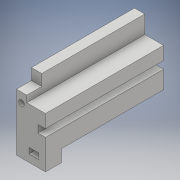
# Autodesk Inventor part: side
Saved by Autodesk Inventor 2018 (Build 220112000, 112)
## iProperties
Created: 2018-05-15
Part Number: side
Material: Generic
Document SubType Name: Modeling
Designer: bitbots
Density: 1 g/cm^3
Appearance: Default
Author: bitbots
Autodesk Inventor part; units mm, degrees
ref_plane "YZ Plane" through (0, 0, 0) normal (1, 0, 0) x (0, 1, 0)
ref_plane "XZ Plane" through (0, 0, 0) normal (0, 1, 0) x (-1, 0, 0)
ref_plane "XY Plane" through (0, 0, 0) normal (0, 0, 1) x (1, 0, 0)
ref_plane "Work Plane1" through (0, 0, 0) normal (0, 0, 1) x (1, 0, 0)
sketch "Sketch1" plane through (0, 0, 0) normal (0, 0, 1) x (1, 0, 0)
  circle A0 centre (-17.3, 4) radius 1.35 projected
  circle A1 centre (-17.3, -18) radius 1.35 projected
  circle A2 centre (-17.3, -40) radius 1.35 projected
  line L0 (-17.3, 4) -> (-14.8, 4)
  line L1 (-14.8, 4) -> (-14.8, 9)
  line L2 (-14.8, 9) -> (-20.3, 9)
  line L3 (-17.3, -40) -> (-17.3, -54)
  line L4 (-14.8, 4) -> (-14.8, -54)
  line L5 (-14.8, -54) -> (-17.3, -54)
  line L6 (-17.3, -54) -> (-20.3, -54)
  line L7 (-20.3, -54) -> (-20.3, 9)
  point P0 (0, 0)
  dimension "d0" = 2.5
  dimension "d1" = 5
  dimension "d2" = 5.5
  dimension "d3" = 14
  constraints: 16 end point, 3 perpendicular, 2 horizontal, 1 parallel, 1 point on line, 1 vertical
  measures "d0" distance of L0.start L0.end
  measures "d1" distance of L0.end L1.end
  measures "d2" distance of L1.end L2.end
  measures "d3" distance of L3.start L3.end
extrude "Extrusion1" add sketch "Sketch1" along normal blind 36.5
sketch "Sketch2" plane through (-20.3, -54, 0) normal (0, -1, 0) x (1, 0, 0)
  line L0 (0, 0) -> (5.5, 0) projected
  line L1 (5.5, 0) -> (5.5, 36.5) projected
  line L2 (0, 36.5) -> (5.5, 36.5) projected
  line L3 (0, 0) -> (0, 36.5) projected
  line L4 (2.75, 36.5) -> (2.75, 25.5)
  circle A0 centre (2.75, 25.5) radius 1.5
  point P0 (20.3, 0)
  dimension "d6" = 11
  dimension "d7" = 3
  constraints: 2 end point, 1 centre point, 1 coincident, 1 midpoint, 1 vertical
  measures "d6" distance of L4.start L4.end
  measures "d7" diameter of A0
extrude "Extrusion2" cut sketch "Sketch2" against normal blind 10 contours A0
sketch "Sketch3" plane through (-20.3, -54, 0) normal (-1, 0, 0) x (0, 0, 1)
  line L0 (0, 63) -> (0, 0) projected
  line L1 (0, 0) -> (36.5, 0) projected
  line L2 (36.5, 63) -> (36.5, 0) projected
  line L3 (0, 63) -> (36.5, 63) projected
  line L4 (0, 0) -> (36.5, 0) projected
  line L5 (36.5, 0) -> (28.5, 0)
  line L6 (28.5, 0) -> (28.5, 8)
  line L7 (28.5, 8) -> (36.5, 8)
  line L8 (36.5, 8) -> (36.5, 0)
  point P0 (0, 54)
  dimension "d10" = 8
  dimension "d11" = 8
  constraints: 8 end point, 2 parallel, 1 horizontal, 1 perpendicular
  measures "d10" distance of L6.end L7.end
  measures "d11" distance of L5.end L6.end
extrude "Extrusion3" cut sketch "Sketch3" against normal blind 10 contours L6 L7 L2 L1
sketch "Sketch4" plane through (-20.3, 9, 0) normal (0, 1, 0) x (1, 0, 0)
  line L0 (5.5, 0) -> (0, 0) projected
  line L1 (0, 0) -> (0, -36.5) projected
  line L2 (5.5, -36.5) -> (0, -36.5) projected
  line L3 (5.5, 0) -> (5.5, -36.5) projected
  line L4 (6.8, -6) -> (8.8, -6) projected
  line L5 (6.8, -6) -> (5.5, -6)
  line L6 (5.5, -6) -> (5.5, -6.5)
  line L7 (5.5, 0) -> (5.5, -28.5) projected
  line L8 (5.5, -6.5) -> (15.5, -6.5)
  line L9 (15.5, -6.5) -> (15.5, -11.5)
  line L10 (15.5, -11.5) -> (5.5, -11.5)
  line L11 (5.5, -11.5) -> (5.5, -6.5)
  point P0 (20.3, 0)
  dimension "d14" = 0.5
  dimension "d15" = 10
  dimension "d16" = 5
  constraints: 12 end point, 2 parallel, 2 perpendicular, 2 point on line, 1 horizontal
  measures "d14" distance of L5.end L6.end
  measures "d15" distance of L9.end L10.end
  measures "d16" distance of L8.end L9.end
extrude "Extrusion4" add sketch "Sketch4" against normal up to surface (63 mm away) contours L8 L9 L10 L3
sketch "Sketch5" plane through (-4.8, 9, 6.5) normal (0, 0, -1) x (-1, 0, 0)
  circle A0 centre (12.5, -49) radius 1.35 projected
  circle A1 centre (12.5, -27) radius 1.35 projected
  circle A2 centre (12.5, -5) radius 1.35 projected
  line L0 (10, -63) -> (10, 0) projected
  line L1 (15.5, -63) -> (10, -63) projected
  line L2 (15.5, 0) -> (15.5, -63) projected
  line L3 (10, 0) -> (15.5, 0) projected
  line L4 (0, -63) -> (10, -63) projected
  line L5 (10, 0) -> (10, -63) projected
  line L6 (0, 0) -> (10, 0) projected
  line L7 (0, 0) -> (0, -63) projected
  line L8 (-19.8, 5.5) -> (-16.3, 5.5) projected
  line L9 (-19.8, 5.5) -> (-24.9, -0.5) projected
  line L10 (-24.9, -0.5) -> (-24.9, -53.6) projected
  line L11 (-24.9, -53.6) -> (-19.8, -59.6) projected
  line L12 (-19.8, -59.6) -> (10.2, -59.6) projected
  line L13 (10.2, -59.6) -> (15.3, -53.6) projected
  line L14 (15.3, -53.6) -> (15.3, -0.5) projected
  line L15 (15.3, -0.5) -> (10.2, 5.5) projected
  line L16 (6.7, 5.5) -> (10.2, 5.5) projected
  arc A3 (9.7, 2.5) -> (6.7, 5.5) centre (6.7, 2.5) ccw projected
  line L17 (9.7, -51) -> (9.7, 2.5) projected
  arc A4 (6.7, -54) -> (9.7, -51) centre (6.7, -51) ccw projected
  line L18 (-16.3, -54) -> (6.7, -54) projected
  arc A5 (-19.3, -51) -> (-16.3, -54) centre (-16.3, -51) ccw projected
  line L19 (-19.3, 2.5) -> (-19.3, -51) projected
  arc A6 (-16.3, 5.5) -> (-19.3, 2.5) centre (-16.3, 2.5) ccw projected
  circle A7 centre (12.5, -5) radius 1.35 projected
  circle A8 centre (12.5, -27) radius 1.35 projected
  circle A9 centre (12.5, -49) radius 1.35 projected
  circle A10 centre (6.2, -56.8) radius 1.35 projected
  circle A11 centre (-22.1, -5) radius 1.35 projected
  circle A12 centre (-22.1, -27) radius 1.35 projected
  circle A13 centre (-22.1, -49) radius 1.35 projected
  circle A14 centre (-15.8, -56.8) radius 1.35 projected
  line L20 (10, 0) -> (10, -63) projected
  line L21 (10, -63) -> (0, -63)
  line L22 (0, -63) -> (0, -54.5)
  line L23 (0, -54.5) -> (10, -54.5)
  line L24 (10, -54.5) -> (10, -63)
  point P0 (-4.8, -9)
  dimension "d19" = 10
  dimension "d20" = 8.5
  constraints: 8 end point, 2 parallel, 1 horizontal, 1 perpendicular
  measures "d19" distance of L22.end L23.end
  measures "d20" distance of L21.end L22.end
extrude "Extrusion5" add sketch "Sketch5" along normal up to surface (6.5 mm away) contours L0 L12 L7 L23 | L0 L4 L7 L12
ref_plane "Work Plane2" through (0, 0, 4) normal (0, 0, -1) x (-1, 0, 0)
sketch "Sketch6" plane through (0, 0, 4) normal (0, 0, -1) x (-1, 0, 0)
  circle A0 centre (17.3, 4) radius 1.35 projected
  circle A1 centre (17.3, -18) radius 1.35 projected
  circle A2 centre (11, -47.8) radius 1.35 projected
  circle A3 centre (17.3, -40) radius 1.35 projected
  circle A4 centre (17.3, -18) radius 1.35 projected
  circle A5 centre (17.3, 4) radius 1.35 projected
  line L0 (20.3, -54) -> (4.8, -54) projected
  line L1 (20.3, 9) -> (20.3, -54) projected
  line L2 (14.8, 9) -> (20.3, 9) projected
  line L3 (14.8, -45.5) -> (14.8, 9) projected
  line L4 (14.8, -45.5) -> (4.8, -45.5) projected
  line L5 (4.8, -45.5) -> (4.8, -54) projected
  circle A6 centre (11, -47.8) radius 1.35 projected
  circle A7 centre (11, -47.8) radius 1.35 projected
  line L6 (17.3, 4) -> (17.3, 6.6)
  line L7 (18.8011, 6.6) -> (20.3022, 4)
  line L8 (20.3022, 4) -> (18.8011, 1.4)
  line L9 (18.8011, 1.4) -> (15.7989, 1.4)
  line L10 (15.7989, 1.4) -> (14.2978, 4)
  line L11 (14.2978, 4) -> (15.7989, 6.6)
  line L12 (15.7989, 6.6) -> (18.8011, 6.6)
  line L13 (18.8011, 1.4) -> (28.5961, 1.4)
  line L14 (28.5961, 1.4) -> (28.5961, 6.6)
  line L15 (28.5961, 6.6) -> (18.8011, 6.6)
  line L16 (18.8011, 6.6) -> (18.8011, 1.4)
  line L17 (11, -47.8) -> (13.6, -47.8)
  line L18 (13.6, -49.3011) -> (11, -50.8022)
  line L19 (11, -50.8022) -> (8.4, -49.3011)
  line L20 (8.4, -49.3011) -> (8.4, -46.2989)
  line L21 (8.4, -46.2989) -> (11, -44.7978)
  line L22 (11, -44.7978) -> (13.6, -46.2989)
  line L23 (13.6, -46.2989) -> (13.6, -49.3011)
  line L24 (13.6, -49.3011) -> (8.4, -49.3011)
  line L25 (8.4, -49.3011) -> (8.4, -56.2377)
  line L26 (8.4, -56.2377) -> (13.6, -56.2377)
  line L27 (13.6, -56.2377) -> (13.6, -49.3011)
  line L28 (18.8011, -15.4) -> (20.3022, -18)
  line L29 (20.3022, -18) -> (18.8011, -20.6)
  line L30 (18.8011, -20.6) -> (28.5961, -20.6)
  line L31 (28.5961, -20.6) -> (28.5961, -15.4)
  line L32 (28.5961, -15.4) -> (18.8011, -15.4)
  line L33 (18.8011, -15.4) -> (18.8011, -20.6)
  line L34 (17.3, -18) -> (17.3, -15.4)
  line L35 (18.8011, -20.6) -> (15.7989, -20.6)
  line L36 (15.7989, -15.4) -> (18.8011, -15.4)
  line L37 (15.7989, -20.6) -> (14.2978, -18)
  line L38 (14.2978, -18) -> (15.7989, -15.4)
  line L39 (18.8011, -37.4) -> (20.3022, -40)
  line L40 (20.3022, -40) -> (18.8011, -42.6)
  line L41 (18.8011, -42.6) -> (28.5961, -42.6)
  line L42 (28.5961, -42.6) -> (28.5961, -37.4)
  line L43 (28.5961, -37.4) -> (18.8011, -37.4)
  line L44 (18.8011, -37.4) -> (18.8011, -42.6)
  line L45 (17.3, -40) -> (17.3, -37.4)
  line L46 (18.8011, -42.6) -> (15.7989, -42.6)
  line L47 (15.7989, -37.4) -> (18.8011, -37.4)
  line L48 (15.7989, -42.6) -> (14.2978, -40)
  line L49 (14.2978, -40) -> (15.7989, -37.4)
  point P0 (0, 0)
  dimension "d24" = 2.6
  dimension "d25" = 2.6
  dimension "d28" = 22
  constraints: 88 end point, 4 coincident, 4 parallel, 3 horizontal, 2 midpoint, 2 perpendicular, 2 vertical, 72 other
  measures "d24" distance of L6.start L6.end
  measures "d25" distance of L17.start L17.end
  measures "d28" distance of L7.start L28.start
extrude "Extrusion6" cut sketch "Sketch6" against normal blind 3 contours A2 | L27 L26 L25 L0 | L0 L25 L19 L18 L27 | L41 L40 L1 | L1 L43 L42 L41 | L24 L20 L21 L4 L22 L23 | L18 L19 L24 | L39 L43 L1 | L40 L44 L39 | L46 L48 L3 L49 L47 L44 | L30 L29 L1 | L1 L32 L31 L30 | L48 L49 L3 | L21 L22 L4 | L28 L32 L1 | L29 L33 L28 | L35 L37 L3 L38 L36 L33 | L37 L38 L3 | L13 L8 L1 | L1 L15 L14 L13 | L7 L15 L1 | L8 L16 L7 | L9 L10 L3 L11 L12 L16 | L10 L11 L3
sketch "Sketch7" plane through (0, 0, 36.5) normal (0, 0, 1) x (1, 0, 0)
  line L0 (-20.3, -46) -> (-14.8, -46) projected
  line L1 (-14.8, -46) -> (-14.8, 9) projected
  line L2 (-14.8, 9) -> (-20.3, 9) projected
  line L3 (-20.3, 9) -> (-20.3, -46) projected
  circle A0 centre (-17.3, 4) radius 1.35 projected
  circle A1 centre (-17.3, -18) radius 1.35 projected
  circle A2 centre (-17.3, -40) radius 1.35 projected
  point P0 (0, 0)
extrude "Extrusion7" add sketch "Sketch7" against normal blind 25 contours A0 | A1 | A2
ref_plane "Work Plane3" through (-20.3, -49, 28.5) normal (0, -1, 0) x (1, 0, 0)
sketch "Sketch8" plane through (-20.3, -49, 28.5) normal (0, -1, 0) x (1, 0, 0)
  circle A0 centre (2.75, -3) radius 1.5 projected
  line L0 (2.75, -3) -> (2.75, -0.4)
  line L1 (4.2511, -0.4) -> (5.7522, -3)
  line L2 (5.7522, -3) -> (4.2511, -5.6)
  line L3 (4.2511, -5.6) -> (1.2489, -5.6)
  line L4 (1.2489, -5.6) -> (-0.2522, -3)
  line L5 (-0.2522, -3) -> (1.2489, -0.4)
  line L6 (1.2489, -0.4) -> (4.2511, -0.4)
  line L7 (1.2489, -0.4) -> (-2.7612, -0.4)
  line L8 (-2.7612, -0.4) -> (-2.7612, -5.6)
  line L9 (-2.7612, -5.6) -> (1.2489, -5.6)
  line L10 (1.2489, -5.6) -> (1.2489, -0.4)
  point P0 (20.3, -28.5)
  dimension "d38" = 2.6
  constraints: 22 end point, 2 parallel, 1 coincident, 1 horizontal, 1 midpoint, 1 perpendicular, 1 vertical, 13 other
  measures "d38" distance of L0.start L0.end
extrude "Extrusion8" cut sketch "Sketch8" against normal blind 3 contours A0 L0 L6 L1 L2 L3 L10 | A0 L10 L6 L0 | L10 L4 L5 | L9 L8 L7 L5 L4
sketch "Sketch9" plane through (-20.3, 9, 0) normal (0, 1, 0) x (1, 0, 0)
  line L0 (5.5, 0) -> (0, 0) projected
  line L1 (0, 0) -> (0, -36.5) projected
  line L2 (5.5, -36.5) -> (0, -36.5) projected
  line L3 (5.5, -11.5) -> (5.5, -36.5) projected
  line L4 (5.5, -11.5) -> (15.5, -11.5) projected
  line L5 (15.5, -11.5) -> (15.5, -6.5) projected
  line L6 (15.5, -6.5) -> (5.5, -6.5) projected
  line L7 (5.5, 0) -> (5.5, -6.5) projected
  line L8 (5.5, -11.5) -> (15.5, -11.5) projected
  line L9 (5.5, -11.5) -> (5.5, -28.5) projected
  line L10 (15.5, -11.5) -> (5.5, -11.5)
  line L11 (5.5, -20) -> (15.5, -20)
  line L12 (5.5, -20) -> (11.5, -20)
  line L13 (5.5, -24) -> (5.5, -20)
  line L14 (15.5, -24) -> (15.5, -27)
  line L15 (15.5, -27) -> (5.5, -27)
  line L16 (5.5, -27) -> (5.5, -24)
  line L17 (5.5, -11.5) -> (15.5, -11.5)
  line L18 (15.5, -11.5) -> (15.5, -16)
  line L19 (15.5, -16) -> (5.5, -16)
  line L20 (5.5, -16) -> (5.5, -11.5)
  line L21 (5.5, -16) -> (11.5, -16)
  line L22 (11.5, -16) -> (11.5, -20)
  line L23 (11.5, -20) -> (5.5, -20)
  line L24 (5.5, -20) -> (5.5, -16)
  line L25 (5.5, -20) -> (15.5, -20)
  line L26 (15.5, -20) -> (15.5, -27)
  line L27 (15.5, -27) -> (5.5, -27)
  line L28 (5.5, -27) -> (5.5, -20)
  point P0 (20.3, 0)
  dimension "d41" = 8.5
  dimension "d44" = 10
  dimension "d45" = 3
  dimension "d48" = 4.5
  constraints: 38 end point, 8 parallel, 5 horizontal, 3 perpendicular, 1 midpoint
  measures "d41" distance of L11.start L10.end
  measures "d44" distance of L14.end L15.end
  measures "d45" distance of L14.start L14.end
  measures "d48" distance of L17.end L18.end
extrude "Extrusion9" add sketch "Sketch9" against normal up to surface (63 mm away) contours L18 L19 L3 L4 | L3 L11 L26 L14 L15 | L19 L22 L11 L3
sketch "Sketch11" plane through (-20.3, -54, 28.5) normal (0, 0, 1) x (1, 0, 0)
  line L0 (5.5, 8) -> (5.5, 0) projected
  line L1 (0, 8) -> (5.5, 8) projected
  line L2 (0, 0) -> (0, 8) projected
  line L3 (5.5, 0) -> (0, 0) projected
  point P0 (20.3, 54)
extrude "Extrusion10" add sketch "Sketch11" along normal blind 2
body "Solid1"
